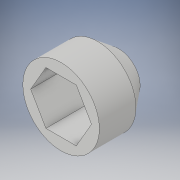
# Autodesk Inventor part: mouthcover
Saved by Autodesk Inventor 2019 (Build 230136000, 136)
## iProperties
Created: 2020-09-18
Part Number: mouthcover
Material: Generic
Document SubType Name: Modeling
Designer: ASUS
Density: 1 g/cm^3
Appearance: Default
Author: ASUS
Autodesk Inventor part; units mm, degrees
ref_plane "YZ Plane" through (0, 0, 0) normal (1, 0, 0) x (0, 1, 0)
ref_plane "XZ Plane" through (0, 0, 0) normal (0, 1, 0) x (-1, 0, 0)
ref_plane "XY Plane" through (0, 0, 0) normal (0, 0, 1) x (1, 0, 0)
sketch "Sketch1" plane through (0, 0, 0) normal (0, 0, 1) x (1, 0, 0)
  circle A0 centre (0, 0) radius 4.5
  dimension "d0" = 9
  constraints: 1 centre point, 1 coincident
  measures "d0" diameter of A0
extrude "Extrusion1" add sketch "Sketch1" along normal blind 6.8
sketch "Sketch2" plane through (0, 0, 6.8) normal (0, 0, 1) x (1, 0, 0)
  line L0 (-1.7898, 3.1) -> (1.7898, 3.1)
  line L1 (1.7898, 3.1) -> (3.5796, 0)
  line L2 (3.5796, 0) -> (1.7898, -3.1)
  line L3 (1.7898, -3.1) -> (-1.7898, -3.1)
  line L4 (-1.7898, -3.1) -> (-3.5796, 0)
  line L5 (-3.5796, 0) -> (-1.7898, 3.1)
  point P0 (0, 0)
  point P1 (0, 3.1)
  point P2 (0, -3.1)
  dimension "d3" = 6.2
  dimension "d4" = 6.2
  constraints: 12 end point, 5 equal length, 2 midpoint, 2 vertical alignment, 1 horizontal, 1 horizontal alignment, 1 parallel
  measures "d3" distance between parallel lines of L3 L0
  measures "d4" distance between parallel lines of L2 L5
extrude "Extrusion2" cut sketch "Sketch2" against normal blind 5.3
sketch "Sketch3" plane through (0, 0, 0) normal (0, 0, -1) x (-1, 0, 0)
  circle A0 centre (0, 0) radius 1.25
  dimension "d7" = 2.5
  constraints: 1 centre point, 1 coincident
  measures "d7" diameter of A0
sketch "Sketch4" plane through (0, 0, 1.5) normal (0, 0, 1) x (1, 0, 0)
  circle A0 centre (0, 0) radius 3.1
  dimension "d8" = 6.2
  constraints: 1 centre point, 1 coincident
  measures "d8" diameter of A0
loft "Loft1" cut profiles "Sketch4", "Sketch3"
sketch "Sketch5" plane through (0, 0, 0) normal (0, 1, 0) x (-1, 0, 0)
  line L0 (-4.5, 0) -> (4.5, 0) projected
  line L1 (2.5, 0) -> (4.5, 2.5)
  line L2 (4.5, 2.5) -> (4.5, 0)
  line L3 (4.5, 0) -> (2.5, 0)
  line L4 (0, -0.5) -> (0, 3) projected
  point P0 (0, 0)
  dimension "d14" = 2.5
  dimension "d15" = 2
  constraints: 6 end point, 1 collinear, 1 perpendicular, 1 point on line
  measures "d14" distance of L1.end L0.end
  measures "d15" distance of L1.start L0.end
revolve "Revolution1" cut sketch "Sketch5" angle 360 about axis through (0, 0, -10) along (0, 0, 1)
equation "\"d4\" = d3"
body "Solid1"
